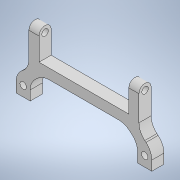
# Autodesk Inventor part: Стойка для камеры
Saved by Autodesk Inventor 2020 (Build 240168000, 168)
## iProperties
Created: 2021-04-12
Part Number: Стойка для камеры
Material: Типовые
Document SubType Name: Обычные детали
Designer: Антон
Density: 1 g/cm^3
Appearance: По умолчанию
Sheet Metal Rule: По умолчанию
Author: Антон
Autodesk Inventor part; units mm, degrees
ref_plane "YZ Plane" through (0, 0, 0) normal (1, 0, 0) x (0, 1, 0)
ref_plane "XZ Plane" through (0, 0, 0) normal (0, 1, 0) x (-1, 0, 0)
ref_plane "XY Plane" through (0, 0, 0) normal (0, 0, 1) x (1, 0, 0)
sketch "Эскиз1" plane through (0, 0, 0) normal (0, 0, 1) x (1, 0, 0)
  line L0 (0, 0) -> (5, 0)
  line L1 (5, 0) -> (5, 7)
  line L2 (5, 7) -> (0, 7)
  line L3 (0, 7) -> (0, 0)
  line L4 (0, 0) -> (27.2, 0)
  line L5 (27.2, 0) -> (27.2, -5)
  line L6 (27.2, -5) -> (0, -5)
  line L7 (0, -5) -> (0, 0)
  dimension "d0" = 5
  dimension "d1" = 7
  dimension "d2" = 27.2
  dimension "d3" = 5
  constraints: 16 end point, 4 parallel, 2 horizontal, 2 perpendicular
  measures "d0" distance of L2.end L1.end
  measures "d1" distance of L1.end L0.end
  measures "d2" distance of L5.end L6.end
  measures "d3" distance of L4.end L5.end
extrude "Выдавливание1" add sketch "Эскиз1" along normal blind 6
sketch "Эскиз4" plane through (0, 7, 0) normal (0, 1, 0) x (1, 0, 0)
  line L0 (0, 0) -> (0, -6) projected
  line L1 (0, 0) -> (0, -6) projected
  line L2 (5, 0) -> (0, 0) projected
  line L3 (0, 0) -> (0, -6) projected
  line L4 (5, -6) -> (0, -6) projected
  line L5 (5, 0) -> (5, -6) projected
  point P0 (0, -6)
  point P1 (0, 0)
extrude "Выдавливание2" add sketch "Эскиз4" along normal blind 7.2
fillet "Сопряжение1" radius 3 2 edges at (2.5, 14.2, 6) (2.5, 14.2, 0)
sketch "Эскиз5" plane through (5, 0, 6) normal (1, 0, 0) x (0, 0, -1)
  line L0 (0, -5) -> (0, -5) projected
  arc A0 (6, 11.2) -> (0, 11.2) centre (3, 11.2) ccw projected
  point P0 (6, 0)
  point P1 (6, -5)
  point P2 (2.5, 25.2)
  constraints: 2 other
hole "Отверстие2" at (5, 11.2, 3) direction (-1, 0, 0) diameter 3.2 depth 5
mirror "Зеркальное отражение1" about plane through (27.2, -5, 0) normal (1, 0, 0)
sketch "Эскиз9" plane through (0, 0, 0) normal (0, 0, -1) x (-1, 0, 0)
  line L0 (0, -5) -> (-54.4, -5) projected
  line L1 (-54.4, 11.2) -> (-54.4, -5) projected
  line L2 (-54.4, -5) -> (-60.75, -10.3)
  line L3 (-60.75, -10.3) -> (-60.75, -18.8)
  line L4 (-60.75, -18.8) -> (-53.75, -18.8)
  line L5 (-53.75, -18.8) -> (-53.75, -10.3)
  line L6 (-53.75, -10.3) -> (-47.4, -5)
  point P0 (0, 0)
  dimension "d82" = 13.8
  dimension "d83" = 7
  dimension "d86" = 8.5
  dimension "d94" = 6.35
  constraints: 10 end point, 4 parallel, 2 perpendicular
  measures "d82" distance between parallel lines of L0 L4
  measures "d83" distance between parallel lines of L5 L3
  measures "d86" distance from line of L5.end L4
  measures "d94" distance between parallel lines of L1 L3
extrude "Выдавливание4" add sketch "Эскиз9" against normal blind 6
sketch "Эскиз11" plane through (0, 0, 6) normal (0, 0, 1) x (1, 0, 0)
  line L0 (57.25, -18.8) -> (57.25, -13.85)
  line L1 (53.75, -18.8) -> (60.75, -18.8) projected
  point P0 (0, 0)
  dimension "d91" = 4.95
  constraints: 2 end point, 1 midpoint, 1 perpendicular
  measures "d91" distance of L0.start L0.end
hole "Отверстие6" at (57.25, -13.85, 6) direction (0, 0, -1) diameter 3.2 end through all
ref_plane "РабПлоскость1" through (27.2, 11.2, 3) normal (1, 0, 0) x (0, 0, -1)
mirror "Зеркальное отражение2" about plane through (27.2, 11.2, 3) normal (1, 0, 0) of "Выдавливание4", "Отверстие6"
fillet "Сопряжение3" radius 8 8 edges at (60.75, -10.3, 3) (53.75, -10.3, 3) (0.65, -10.3, 3) (-6.35, -10.3, 3) (0, -5, 3) (7, -5, 3) (47.4, -5, 3) (54.4, -5, 3)
equation "\"Радиус_гибки\" = Толщина"
equation "\"Ширина_просечки\" = Толщина"
equation "\"Глубина_просечки\" = 0.5 * Толщина"
equation "\"Размер_просечки\" = 4 * Толщина"
equation "\"Мин_остаток\" = 2 * Толщина"
equation "\"Радиус_перехода\" = Радиус_гибки"
equation "\"Радиус_Якоби\" = Толщина"
equation "\"Размер_зазора\" = Толщина"
equation "\"Толщина\" = 0.5"
